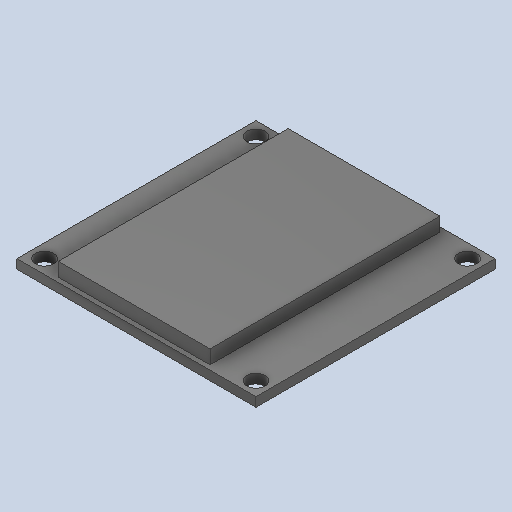
# Autodesk Inventor part: Screen
Saved by Autodesk Inventor 2025.2 (Build 292293000, 293)
## iProperties
Created: 2024-03-12
Part Number: Screen
Material: Generic
Document SubType Name: Modeling
Designer: mirun
Density: 1 g/cm^3
Appearance: Default
Author: mirun
Autodesk Inventor part; units mm, degrees
ref_plane "YZ Plane" through (0, 0, 0) normal (1, 0, 0) x (0, 1, 0)
ref_plane "XZ Plane" through (0, 0, 0) normal (0, 1, 0) x (-1, 0, 0)
ref_plane "XY Plane" through (0, 0, 0) normal (0, 0, 1) x (1, 0, 0)
sketch "Sketch1" plane through (0, 0, 0) normal (0, 1, 0) x (-1, 0, 0)
  line L0 (-13, 13) -> (13, 13)
  line L1 (13, 13) -> (13, -13)
  line L2 (13, -13) -> (-13, -13)
  line L3 (-13, -13) -> (-13, 13)
  line L4 (-13, 13) -> (13, -13) construction
  line L5 (13, 13) -> (-13, -13) construction
  circle A0 centre (11.5, 11.5) radius 1
  line L6 (0, 0) -> (3.4228, 0) construction
  line L7 (0, 0) -> (0, 5.3357) construction
  circle A1 centre (11.5, -11.5) radius 1
  circle A2 centre (-11.5, 11.5) radius 1
  circle A3 centre (-11.5, -11.5) radius 1
  dimension "d0" = 26
  dimension "d1" = 26
  dimension "d2" = 2
  dimension "d3" = 1.5
  constraints: 16 end point, 4 centre point, 3 symmetric about line, 2 horizontal, 2 midpoint, 2 parallel, 1 perpendicular, 1 point on line, 1 vertical, 3 other
  measures "d0" distance of L1.end L2.end
  measures "d1" distance of L0.end L1.end
  measures "d2" diameter of A0
  measures "d3" distance from line of L1 A0.centre
extrude "Extrusion1" add sketch "Sketch1" along normal blind 1
sketch "Sketch2" plane through (0, 1, 0) normal (0, 1, 0) x (1, 0, 0)
  line L0 (-13, 13) -> (-13, -13) construction
  line L1 (0, 0) -> (-10.4427, 0) construction
  line L2 (7.5, -12.5) -> (-9, -12.5)
  line L3 (-9, -12.5) -> (-9, 12.5)
  line L4 (-9, 12.5) -> (7.5, 12.5)
  line L5 (7.5, 12.5) -> (7.5, -12.5)
  line L6 (7.5, -12.5) -> (-9, 12.5) construction
  line L7 (-9, -12.5) -> (7.5, 12.5) construction
  point P0 (-0.75, 0)
  dimension "d6" = 16.5
  dimension "d7" = 25
  dimension "d8" = 4
  constraints: 14 end point, 2 horizontal, 2 midpoint, 2 parallel, 1 perpendicular, 1 point on line
  measures "d6" distance of L3.end L4.end
  measures "d7" distance of L2.end L3.end
  measures "d8" distance between parallel lines of L3 L0
extrude "Extrusion2" add sketch "Sketch2" along normal blind 1.5
body "Solid1"
